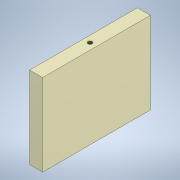
# Autodesk Inventor part: Paddle
Saved by Autodesk Inventor 2020 (Build 240168000, 168)
## iProperties
Created: 2020-06-22
Part Number: Paddle
Material: Polypropylene
Document SubType Name: Modeling
Designer: Bruno
Density: 0.899 g/cm^3
Appearance: Smooth - Ash
Author: Bruno
Autodesk Inventor part; units mm, degrees
ref_plane "YZ Plane" through (0, 0, 0) normal (1, 0, 0) x (0, 1, 0)
ref_plane "XZ Plane" through (0, 0, 0) normal (0, 1, 0) x (-1, 0, 0)
ref_plane "XY Plane" through (0, 0, 0) normal (0, 0, 1) x (1, 0, 0)
sketch "Sketch1" plane through (0, 0, 0) normal (0, 0, 1) x (1, 0, 0)
  line L0 (0, 0) -> (10, 0)
  line L1 (10, 0) -> (10, 63)
  line L2 (10, 63) -> (0, 63)
  line L3 (0, 63) -> (0, 0)
  dimension "d0" = 10
  dimension "d1" = 63
  constraints: 8 end point, 2 parallel, 1 horizontal, 1 perpendicular
  measures "d0" distance of L2.end L1.end
  measures "d1" distance of L1.end L0.end
extrude "Extrusion1" add sketch "Sketch1" along normal blind 82.8
sketch "m" plane through (0, 63, 0) normal (0, 1, 0) x (1, 0, 0)
  line L0 (0, 0) -> (0, -82.8) projected
  line L1 (10, 0) -> (0, 0) projected
  point P0 (5, -41.4)
  dimension "d4" = 5
  dimension "d5" = 41.4
  measures "d4" distance from line of L0 point (5, -41.4)
  measures "d5" distance from line of L1 point (5, -41.4)
hole "Hole1" at (5, 63, 41.4) direction (0, -1, 0) diameter 3.242 depth 12 tip angle 118 thread size "M4x0.7" class "6H" standard "ISO Metric profile"
equation "\"d5\" = 0.5 * d2"
equation "\"d2\" = 82.8"
body "Solid1"
